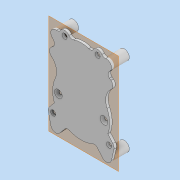
# Autodesk Inventor part: base-lidar
Saved by Autodesk Inventor 2022 (Build 260153000, 153)
## iProperties
Created: 2022-07-30
Part Number: base-lidar
Material: Générique
Document SubType Name: Modeling
Designer: andre
Density: 1 g/cm^3
Appearance: Par défaut
Author: andre
Autodesk Inventor part; units mm, degrees
ref_plane "YZ Plane" through (0, 0, 0) normal (1, 0, 0) x (0, 1, 0)
ref_plane "XZ Plane" through (0, 0, 0) normal (0, 1, 0) x (-1, 0, 0)
ref_plane "Plan de construction1" through (0, -197.8162, 0) normal (0, 0, 1) x (-1, 0, 0)
sketch "Esquisse1" plane through (0, -197.8162, 0) normal (0, 0, 1) x (-1, 0, 0)
  arc A0 (-23.6268, -23.8975) -> (-20.477, -9.3243) centre (-31.8353, -14.4963) ccw
  arc A1 (-23.6268, -23.8975) -> (-23.507, -30.0242) centre (-20.996, -26.9106) ccw
  arc A2 (-22.0658, -35.1912) -> (-22.4423, -30.8828) centre (-24.3256, -33.2181) ccw
  line L0 (-22.4423, -30.8828) -> (-23.507, -30.0242)
  line L1 (-23.0131, -36.2761) -> (-22.0658, -35.1912)
  arc A3 (-23.0131, -36.2761) -> (-19.3537, -42.8544) centre (-20, -38.907) ccw
  line L2 (-16.9711, -41.5196) -> (-16.9869, -41.5378)
  arc A4 (-6.0453, -42.9227) -> (6.0453, -42.9227) centre (0, -26.5) ccw
  arc A5 (11.4655, -39.7206) -> (11.4485, -39.7351) centre (13.4112, -42.0041) ccw
  line L3 (16.9869, -41.5378) -> (16.9711, -41.5196)
  arc A6 (19.3537, -42.8544) -> (23.0131, -36.2761) centre (20, -38.907) ccw
  line L4 (21.6977, -34.7696) -> (23.0131, -36.2761)
  arc A7 (21.984, -30.5365) -> (21.6977, -34.7696) centre (23.9573, -32.7962) ccw
  line L5 (23.6265, -29.1024) -> (21.984, -30.5365)
  arc A8 (23.6265, -29.1024) -> (23.5067, -22.9757) centre (20.9956, -26.0893) ccw
  arc A9 (20.4202, -9.4479) -> (23.5067, -22.9757) centre (30.5395, -14.2551) ccw
  arc A10 (20.4202, -9.4479) -> (21.1202, 7.7581) centre (0, 0) ccw
  arc A11 (23.898, 24.583) -> (16.9438, 26.2661) centre (20, 23.6854) ccw
  line L6 (12.7634, 21.3154) -> (16.9438, 26.2661)
  arc A12 (9.2394, 20.5155) -> (12.7634, 21.3154) centre (10.4713, 23.2509) ccw
  arc A13 (9.2394, 20.5155) -> (1.6496, 22.4394) centre (0, 0) ccw
  arc A14 (-2.028, 22.4084) -> (-9.2394, 20.5155) centre (0, 0) ccw
  arc A15 (-12.7634, 21.3154) -> (-9.2394, 20.5155) centre (-10.4713, 23.2509) ccw
  line L7 (-16.9438, 26.2661) -> (-12.7634, 21.3154)
  arc A16 (-16.9438, 26.2661) -> (-23.898, 24.583) centre (-20, 23.6854) ccw
  arc A17 (-21.1202, 7.7581) -> (-20.477, -9.3243) centre (0, 0) ccw
  circle A18 centre (-22, 15) radius 2
  circle A19 centre (-13, -42) radius 2
  arc A20 (-16.3537, -44.18) -> (-9.6181, -44.136) centre (-13, -42) ccw
  arc A21 (-6.0453, -42.9227) -> (-9.6181, -44.136) centre (-7.0816, -45.738) ccw
  arc A22 (-16.3537, -44.18) -> (-19.3537, -42.8544) centre (-18.8691, -45.815) ccw
  arc A23 (-25.898, 15.8976) -> (-25.0562, 12.4194) centre (-22, 15) ccw
  line L8 (-23.898, 24.583) -> (-25.898, 15.8976)
  line L9 (-25.0562, 12.4194) -> (-21.1202, 7.7581)
  line L10 (0, 0) -> (0, -14.4963)
  circle A24 centre (22, 15) radius 2
  circle A25 centre (13, -42) radius 2
  arc A26 (9.6181, -44.136) -> (16.3537, -44.18) centre (13, -42) ccw
  arc A27 (9.6181, -44.136) -> (6.0453, -42.9227) centre (7.0816, -45.738) ccw
  arc A28 (19.3537, -42.8544) -> (16.3537, -44.18) centre (18.8691, -45.815) ccw
  arc A29 (25.0562, 12.4194) -> (25.898, 15.8976) centre (22, 15) ccw
  line L11 (23.898, 24.583) -> (25.898, 15.8976)
  line L12 (25.0562, 12.4194) -> (21.1202, 7.7581)
  circle A30 centre (-18, 0) radius 1.25
  line L13 (0, 0) -> (-3.231, 0)
  circle A31 centre (18, 0) radius 1.25
  arc A32 (1.6496, 22.4394) -> (-2.028, 22.4084) centre (0, 0) ccw
  point P0 (0, -197.8162)
  dimension "d0" = 4
  dimension "d1" = 4
  dimension "d2" = 8
  dimension "d5" = 3
  dimension "d6" = 3
  dimension "d7" = 8
  dimension "d8" = 22
  dimension "d11" = 2.5
  dimension "d12" = 18
  constraints: 56 point on circle, 33 centre point, 28 end point, 15 symmetric about line, 7 tangent, 5 coincident, 2 point on line, 1 horizontal, 1 parallel, 1 vertical, 7 other
  measures "d0" diameter of A18
  measures "d1" diameter of A19
  measures "d2" diameter of A20
  measures "d5" radius of A21
  measures "d6" radius of A22
  measures "d7" diameter of A23
  measures "d8" horizontal distance of A10.centre A23.centre
  measures "d11" diameter of A30
  measures "d12" distance of A10.centre A30.centre
extrude "Extrusion1" add sketch "Esquisse1" along normal blind 2
sketch "Esquisse2" plane through (0, -197.8162, 0) normal (0, 0, 1) x (-1, 0, 0)
  arc A0 (-23.0131, -36.2761) -> (-19.3537, -42.8544) centre (-20, -38.907) ccw projected
  circle A1 centre (-20, -38.907) radius 4
  circle A2 centre (20, -38.907) radius 4
  circle A3 centre (20, 23.6854) radius 4
  circle A4 centre (-20, 23.6854) radius 4
  point P0 (0, -197.8162)
  point P1 (-23.0131, -36.2761)
  constraints: 3 centre point, 3 other
ref_plane "Plan de construction2" through (-24.996, -225.5017, -12) normal (0, 0, 1) x (1, 0, 0)
extrude "Extrusion2" add sketch "Esquisse2" against normal up to surface (12 mm away)
sketch "Esquisse3" plane through (0, -197.8162, 0) normal (0, 0, -1) x (-1, 0, 0)
  arc A0 (12.7634, -21.3154) -> (9.2394, -20.5155) centre (10.4713, -23.2509) ccw construction
  line L0 (-0.4209, 1.0135) -> (9.2394, -20.5155) construction
  line L1 (-0.4209, 1.0135) -> (4.4805, -22.0494) construction
  arc A1 (-9.2394, -20.5155) -> (9.2394, -20.5155) centre (0, 0) ccw construction
  line L2 (9.2394, -20.5155) -> (4.4805, -22.0494)
  line L3 (3.4647, -17.2699) -> (7.2374, -16.0538)
  line L4 (9.2394, -20.5155) -> (7.2374, -16.0538)
  line L5 (3.4647, -17.2699) -> (4.4805, -22.0494)
  point P0 (0, 197.8162)
  dimension "d17" = 5
  dimension "d18" = 5
  constraints: 12 end point, 2 collinear, 2 point on line, 1 parallel, 1 point on circle
  measures "d17" distance of L0.end L1.end
  measures "d18" distance edge to line of A1 L3
extrude "Extrusion3" add sketch "Esquisse3" along normal blind 7
chamfer "Chanfrein1" distance 1.8 angle 45 2 edges at (19.25, -197.8162, 2) (-16.75, -197.8162, 2)
